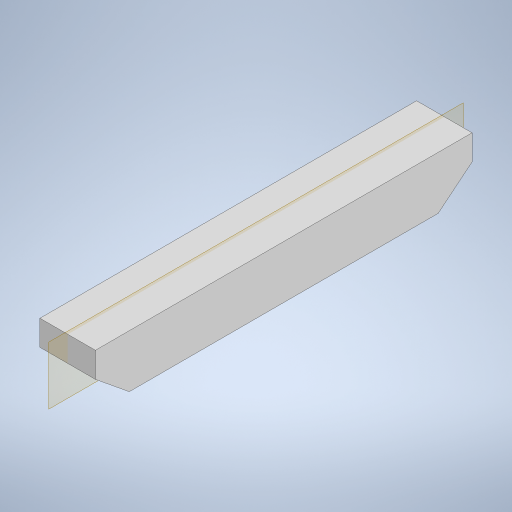
# Autodesk Inventor part: Enemy_Track_collision
Saved by Autodesk Inventor 2024 (Build 280153000, 153)
## iProperties
Created: 2026-05-21
Part Number: Enemy_Track_collision
Material: Generic
Document SubType Name: Modeling
Designer: warny
Density: 1 g/cm^3
Appearance: Default
Author: warny
Autodesk Inventor part; units mm, degrees
ref_plane "XZ Plane" through (0, 0, 0) normal (0, 1, 0) x (-1, 0, 0)
ref_plane "XY Plane" through (0, 0, 0) normal (0, 0, 1) x (1, 0, 0)
sketch "Sketch1" plane through (0, 0, 0) normal (1, 0, 0) x (0, 1, 0)
  line L0 (66.79, 404) -> (66.79, -404)
  line L1 (66.79, -404) -> (12.72, -404)
  line L2 (12.72, -404) -> (-46.497, -331.3)
  line L3 (-46.497, -331.3) -> (-46.497, 331.3)
  line L4 (-46.497, 331.3) -> (12.72, 404)
  line L5 (12.72, 404) -> (66.79, 404)
  point P0 (0, 0)
  dimension "d0" = 331.3
  dimension "d1" = 331.3
  dimension "d2" = 46.497
  dimension "d3" = 46.497
  dimension "d4" = 12.72
  dimension "d5" = 12.72
  dimension "d6" = 404
  dimension "d7" = 404
  dimension "d8" = 66.79
  constraints: 12 end point, 1 parallel, 1 perpendicular, 1 vertical
  measures "d0" vertical distance of L3.end point (0, 0)
  measures "d1" vertical distance of point (0, 0) L2.end
  measures "d2" horizontal distance of L3.end point (0, 0)
  measures "d3" horizontal distance of L2.end point (0, 0)
  measures "d4" horizontal distance of L4.end point (0, 0)
  measures "d5" horizontal distance of L1.end point (0, 0)
  measures "d6" vertical distance of point (0, 0) L4.end
  measures "d7" vertical distance of point (0, 0) L1.end
  measures "d8" horizontal distance of L0.start point (0, 0)
extrude "Extrusion1" add sketch "Sketch1" along normal mid plane 119
body "Solid1"
